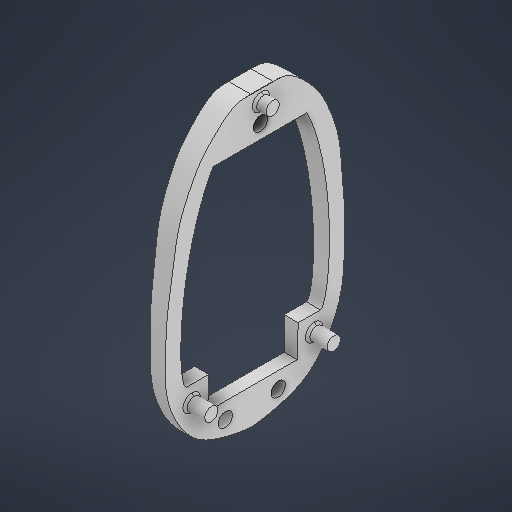
# Autodesk Inventor part: baseplate
Saved by Autodesk Inventor 2026.2 (Build 302298000, 298)
## iProperties
Created: 2026-01-10
Part Number: baseplate
Material: 一般
Document SubType Name: Modeling
Designer: gavin
Density: 1 g/cm^3
Appearance: 預設
Author: gavin
## iProperties of the stored document baseplate_3D 列印.ipt
Created: 2026-01-10
Part Number: baseplate_3D 列印
Material: 一般
Document SubType Name: Modeling
Designer: gavin
Density: 1 g/cm^3
Appearance: 預設
Author: gavin
Autodesk Inventor part; units mm, degrees
ref_plane "YZ Plane" through (0, 0, 0) normal (1, 0, 0) x (0, 1, 0)
ref_plane "XZ Plane" through (0, 0, 0) normal (0, 1, 0) x (-1, 0, 0)
ref_plane "XY Plane" through (0, 0, 0) normal (0, 0, 1) x (1, 0, 0)
sketch "草圖1" plane through (0, 0, 0) normal (1, 0, 0) x (0, 1, 0)
  line L0 (142.8834, -99.6672) -> (-63.4778, -37.9521) construction
  line L1 (-63.4778, -37.9521) -> (21.526, 246.2813) construction
  line L2 (21.526, 246.2813) -> (227.8872, 184.5662) construction
  line L3 (227.8872, 184.5662) -> (142.8834, -99.6672) construction
  line L4 (135.047, -0.0054) -> (0, 0) construction
  spline S0 degree 4 poles (135.047, -0.0054) (135.334, -2.5337) (135.1874, -8.535) (136.3392, -12.217) (120.5543, -27.3688) (113.7441, -30.0248) (99.247, -37.1156) (82.587, -37.7891) (64.9987, -40.7713) (48.9891, -40.2792) (38.159, -40.6834) (24.5334, -37.853) (8.0334, -27.6819) (2.82, -19.3123) (0.1039, -2.6015) (0, 0) knots 0 0 0 0 0 0.115528 0.173115 0.23842 0.313059 0.389931 0.470279 0.548602 0.623865 0.695906 0.765042 0.836544 1 1 1 1 1
  spline S1 degree 4 poles (135.047, -0.0054) (135.3342, 2.5228) (135.1881, 8.5241) (136.3402, 12.206) (120.5565, 27.3591) (113.7465, 30.0156) (99.25, 37.1076) (82.59, 37.7825) (65.002, 40.766) (48.9923, 40.2753) (38.1623, 40.6803) (24.5365, 37.851) (8.0356, 27.6813) (2.8216, 19.3121) (0.1041, 2.6015) (0, 0) knots 0 0 0 0 0 0.115528 0.173115 0.23842 0.313059 0.389931 0.470279 0.548602 0.623865 0.695906 0.765042 0.836544 1 1 1 1 1
  spline S2 degree 4 poles (31.3433, 30.2927) (33.0789, 35.7801) (98.3678, 37.4095) (123.8079, 18.9741) (124.6011, 11.9173) knots 0 0 0 0 0 1 1 1 1 1
  line L5 (124.6011, 11.9173) -> (124.6006, -0.005)
  line L6 (31.3433, 30.2927) -> (31.3429, 20.2239)
  line L7 (31.3429, 20.2239) -> (16.6188, 20.2245)
  line L8 (16.6188, 20.2245) -> (16.618, -0.0007)
  spline S3 degree 4 poles (31.3409, -30.2953) (33.076, -35.7827) (98.3648, -37.4175) (123.8064, -18.984) (124.6001, -11.9273) knots 0 0 0 0 0 1 1 1 1 1
  line L9 (124.6001, -11.9273) -> (124.6006, -0.005)
  line L10 (31.3409, -30.2953) -> (31.3413, -20.2264)
  line L11 (31.3413, -20.2264) -> (16.6172, -20.2258)
  line L12 (16.6172, -20.2258) -> (16.618, -0.0007)
  line L13 (0, 0) -> (25.4836, -0.4448) construction
  point P0 (135.2598, -4.2334)
  point P1 (135.0466, -8.8798)
  point P2 (133.0007, -14.0556)
  point P3 (122.2123, -25.066)
  point P4 (113.4535, -30.3019)
  point P5 (100.5888, -35.3221)
  point P6 (82.7958, -38.1918)
  point P7 (63.7351, -40.1727)
  point P8 (48.5542, -40.4397)
  point P9 (37.6255, -40.0257)
  point P10 (24.8472, -36.9013)
  point P11 (12.8621, -29.8851)
  point P12 (5.8108, -21.5044)
  point P13 (1.2495, -7.9223)
  point P14 (135.2601, 4.2225)
  point P15 (135.0473, 8.8689)
  point P16 (133.0019, 14.0449)
  point P17 (122.2143, 25.0562)
  point P18 (113.4559, 30.2927)
  point P19 (100.5916, 35.314)
  point P20 (82.7989, 38.1851)
  point P21 (63.7384, 40.1675)
  point P22 (48.5574, 40.4358)
  point P23 (37.6288, 40.0227)
  point P24 (24.8502, 36.8993)
  point P25 (12.8645, 29.8841)
  point P26 (5.8126, 21.5039)
  point P27 (1.2502, 7.9222)
  point P28 (46.1532, 33.3798)
  point P29 (100.2162, 26.8889)
  point P30 (121.9838, 16.1061)
  point P31 (46.1505, -33.3835)
  point P32 (100.214, -26.897)
  point P33 (121.9825, -16.116)
  constraints: 21 symmetric about line, 20 end point, 3 perpendicular, 2 point on line, 1 parallel, 44 other
extrude "擠出1" add sketch "草圖1" along normal blind 10
sketch "草圖2" plane through (0, 0, 0) normal (0, 0, 1) x (1, 0, 0)
  line L0 (0, 0) -> (10, 0) projected
  line L1 (0, 135.047) -> (10, 135.047) projected
  line L2 (10, 135.2671) -> (10, 0) projected
  line L3 (10, 135.2671) -> (4.5179, -21.7193)
  point P0 (9.9923, 135.047)
  point P1 (5.2764, 0)
  dimension "d22" = 2
  constraints: 2 end point
  measures "d22" angle of L2 L3
extrude "擠出2" cut sketch "草圖2" along normal mid plane 100 contours L3 L1 L2 L0
sketch "草圖3" plane through (0, 0, 0) normal (-1, 0, 0) x (0, 0, 1)
  line L0 (11.9173, 124.6011) -> (-11.9273, 124.6001) projected
  line L1 (20.2239, 31.3429) -> (30.2927, 31.3433) projected
  line L2 (20.2245, 16.6188) -> (20.2239, 31.3429) projected
  line L3 (-20.2258, 16.6172) -> (20.2245, 16.6188) projected
  line L4 (-20.2264, 31.3413) -> (-20.2258, 16.6172) projected
  line L5 (-30.2953, 31.3409) -> (-20.2264, 31.3413) projected
  circle A0 centre (-0.0052, 129.8238) radius 3
  circle A1 centre (-27.7261, 23.841) radius 3
  circle A2 centre (27.7242, 23.8432) radius 3
  point P0 (-0.005, 124.6006)
  dimension "d25" = 6
  dimension "d26" = 5.2232
  dimension "d27" = 10.4464
  dimension "d28" = 6
  dimension "d29" = 6
  dimension "d30" = 7.5
  dimension "d31" = 7.5
  dimension "d32" = 7.5
  dimension "d33" = 7.5
  constraints: 3 centre point, 1 midpoint, 4 other
  measures "d25" diameter of A0
  measures "d26" distance of point (-0.005, 135.047) A0.centre
  measures "d27" distance of point (-0.005, 124.601) point (-0.005, 135.047)
  measures "d28" diameter of A1
  measures "d29" diameter of A2
  measures "d30" distance from line of L4 A1.centre
  measures "d31" distance from line of A1.centre L5
  measures "d32" distance from line of A2.centre L1
  measures "d33" distance from line of L2 A2.centre
extrude "擠出3" add sketch "草圖3" against normal blind 15
chamfer "倒角1" distance 1 angle 45 3 edges at (9.8099, 129.8238, -3.0052) (6.109, 23.8432, 24.7242) (6.1089, 23.841, -30.7261)
sketch "草圖4" plane through (0, 0, 0) normal (-1, 0, 0) x (0, 0, 1)
  line L0 (11.9173, 124.6011) -> (-11.9273, 124.6001) projected
  spline S0 degree 4 poles (30.2927, 31.3433) (35.7801, 33.0789) (37.4095, 98.3678) (18.9741, 123.8079) (11.9173, 124.6011) knots 0 0 0 0 0 1 1 1 1 1 projected
  line L1 (20.2239, 31.3429) -> (30.2927, 31.3433) projected
  line L2 (20.2245, 16.6188) -> (20.2239, 31.3429) projected
  line L3 (-20.2258, 16.6172) -> (20.2245, 16.6188) projected
  line L4 (-20.2264, 31.3413) -> (-20.2258, 16.6172) projected
  line L5 (-30.2953, 31.3409) -> (-20.2264, 31.3413) projected
  spline S1 degree 4 poles (-11.9273, 124.6001) (-18.984, 123.8064) (-37.4175, 98.3648) (-35.7827, 33.076) (-30.2953, 31.3409) knots 0 0 0 0 0 1 1 1 1 1 projected
  line L6 (-21.198, 114.6005) -> (21.1896, 114.6005)
  point P0 (-3.8131, 114.6005)
  dimension "d40" = 10
  constraints: 2 end point, 1 horizontal, 1 point on line, 6 other
  measures "d40" distance from line of point (-3.813, 114.6) L0
extrude "擠出4" add sketch "草圖4" against normal up to surface contours S0 L6 S1 L0 surface through (9.9923, 135.047, 0) normal (-0.9993908, 0.0348995, 0)
sketch "草圖5" plane through (0, 0, 0) normal (-1, 0, 0) x (0, 0, 1)
  circle A0 centre (-12.0007, 9.1175) radius 3.275
  line L0 (-20.2258, 16.6172) -> (20.2245, 16.6188) projected
  line L1 (0, 0) -> (-0.0007, 16.618) construction
  circle A1 centre (11.9999, 9.1185) radius 3.275
  circle A2 centre (-0.0049, 121.1005) radius 3.275
  line L2 (-21.198, 114.6005) -> (21.1896, 114.6005) projected
  dimension "d43" = 6.55
  dimension "d45" = 7.5
  dimension "d46" = 12
  dimension "d47" = 6.55
  dimension "d48" = 6.5
  constraints: 3 centre point, 2 end point, 1 midpoint, 1 symmetric about line, 1 other
  measures "d43" diameter of A0
  measures "d45" distance from line of A0.centre L0
  measures "d46" horizontal distance of L1.end A0.centre
  measures "d47" diameter of A2
  measures "d48" distance from line of A2.centre L2
extrude "擠出5" cut sketch "草圖5" against normal up to surface surface through (9.9923, 135.047, 0) normal (-0.9993908, 0.0348995, 0)
sketch "草圖6" plane through (0, 0, 0) normal (-1, 0, 0) x (0, 0, 1)
  circle A0 centre (11.9999, 9.1185) radius 3.275 projected
  circle A1 centre (-0.0049, 121.1005) radius 3.275 projected
  circle A2 centre (-12.0007, 9.1175) radius 3.275 projected
  spline S0 degree 4 poles (0, 0) (-2.6015, 0.1039) (-19.3123, 2.82) (-27.6819, 8.0334) (-37.853, 24.5334) (-40.6834, 38.159) (-40.2792, 48.9891) (-40.7713, 64.9987) (-37.7891, 82.587) (-37.1156, 99.247) (-30.0248, 113.7441) (-27.3688, 120.5543) (-12.217, 136.3392) (-8.535, 135.1874) (-2.5337, 135.334) (-0.0054, 135.047) knots 0 0 0 0 0 0.163456 0.234958 0.304094 0.376135 0.451398 0.529721 0.610069 0.686941 0.76158 0.826885 0.884472 1 1 1 1 1 projected
  spline S1 degree 4 poles (-0.0054, 135.047) (2.5228, 135.3342) (8.5241, 135.1881) (12.206, 136.3402) (27.3591, 120.5565) (30.0156, 113.7465) (37.1076, 99.25) (37.7825, 82.59) (40.766, 65.002) (40.2753, 48.9923) (40.6803, 38.1623) (37.851, 24.5365) (27.6813, 8.0356) (19.3121, 2.8216) (2.6015, 0.1041) (0, 0) knots 0 0 0 0 0 0.115528 0.173115 0.23842 0.313059 0.389931 0.470279 0.548602 0.623865 0.695906 0.765042 0.836544 1 1 1 1 1 projected
  line L0 (-21.198, 114.6005) -> (21.1896, 114.6005) projected
  line L1 (20.2239, 31.3429) -> (30.2927, 31.3433) projected
  line L2 (20.2245, 16.6188) -> (20.2239, 31.3429) projected
  line L3 (-20.2258, 16.6172) -> (20.2245, 16.6188) projected
  line L4 (-20.2264, 31.3413) -> (-20.2258, 16.6172) projected
  line L5 (-30.2953, 31.3409) -> (-20.2264, 31.3413) projected
  line L6 (-29.3341, 135.2667) -> (30.2927, 135.2667)
  point P0 (4.9133, 135.2667)
  point P1 (-5.1322, 135.2667)
  constraints: 2 end point, 2 horizontal, 4 other
extrude "擠出6" add sketch "草圖6" against normal up to surface contours L6 S1 S0 surface through (9.9923, 135.047, 0) normal (-0.9993908, 0.0348995, 0)
equation "\"d26\" = 0.5 * d27"
equation "\"d31\" = d30"
equation "\"d32\" = d31"
equation "\"d33\" = d32"
